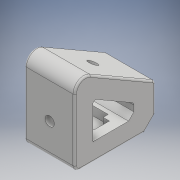
# Autodesk Inventor part: triangle_jig
Saved by Autodesk Inventor 2017 (Build 210142000, 142)
## iProperties
Part Number: triangle_jig
Material: 一般
Document SubType Name: Modeling
Designer: taige
Density: 1 g/cm^3
Appearance: 既定
Author: taige
Autodesk Inventor part; units mm, degrees
ref_plane "YZ Plane" through (0, 0, 0) normal (1, 0, 0) x (0, 1, 0)
ref_plane "XZ Plane" through (0, 0, 0) normal (0, 1, 0) x (-1, 0, 0)
ref_plane "XY Plane" through (0, 0, 0) normal (0, 0, 1) x (1, 0, 0)
sketch "スケッチ1" plane through (0, 0, 0) normal (1, 0, 0) x (0, 1, 0)
  line L0 (-20, 24) -> (63.1384, 24)
  line L1 (63.1384, 24) -> (63.1384, -24)
  line L2 (25, -24) -> (-20, -24)
  line L3 (-20, -24) -> (-20, 24)
  line L4 (-20, 24) -> (63.1384, -24)
  line L5 (-20, -24) -> (25, -24)
  line L6 (25, -24) -> (25, -1.9808)
  line L7 (25, 24) -> (-20, 24)
  line L8 (-20, 24) -> (-20, -24)
  point P0 (0, 0)
  dimension "d6" = 24
  dimension "d7" = 48
  dimension "d96" = 45
  dimension "d98" = 83.1384
  constraints: 18 end point, 4 parallel, 2 horizontal, 2 perpendicular, 2 point on line
  measures "d6" distance from line of point (0, 0) L0
  measures "d7" distance of L2.end L0.start
  measures "d96" distance of L7.end L7.start
  measures "d98" distance of L0.start L0.end
extrude "押し出し1" add sketch "スケッチ1" along normal blind 28 contours L4 L6 L2 L3
sketch "スケッチ2" plane through (28, 0, 0) normal (1, 0, 0) x (0, 0, -1)
  line L0 (-6.6795, -10) -> (14, -10)
  line L1 (14, -10) -> (14, 25.8179)
  line L2 (14, 25.8179) -> (-6.6795, 25.8179)
  line L3 (-6.6795, 25.8179) -> (-6.6795, 13)
  line L4 (-24, -20) -> (24, -20) projected
  line L5 (24, -20) -> (24, 25) projected
  line L6 (-6.6795, -10) -> (14, 25.8179)
  line L7 (14, -10) -> (-6.679, -10)
  line L8 (-6.679, -10) -> (-6.679, 13)
  line L9 (6.5996, 13) -> (14, 13)
  line L10 (14, 13) -> (14, -10)
  point P0 (0, 0)
  point P1 (24, 63.1384)
  dimension "d10" = 20.6795
  dimension "d11" = 35.8179
  dimension "d12" = 10
  dimension "d13" = 10
  dimension "d19" = 20.679
  dimension "d75" = 23
  constraints: 18 end point, 4 parallel, 2 horizontal, 2 perpendicular, 2 point on line
  measures "d10" distance of L2.end L1.end
  measures "d11" distance of L1.end L0.end
  measures "d12" distance between parallel lines of L0 L4
  measures "d13" distance between parallel lines of L5 L1
  measures "d19" distance of L8.end L9.end
  measures "d75" distance between parallel lines of L9 L0
extrude "押し出し2" cut sketch "スケッチ2" against normal blind 40 contours L6 L9 L1 L0
sketch "スケッチ3" plane through (28, -10, 6.6795) normal (0, 1, 0) x (1, 0, 0)
  line L0 (0, 20.6795) -> (0, 0) projected
  line L1 (0, 20.6795) -> (-28, 20.6795) projected
  line L2 (-19.1, 5.5795) -> (-8.9, 5.5795)
  line L3 (-8.9, 5.5795) -> (-8.9, 19.7795)
  line L4 (-8.9, 19.7795) -> (-19.1, 19.7795)
  line L5 (-19.1, 19.7795) -> (-19.1, 5.5795)
  line L6 (-22.6, 8.4295) -> (-5.4, 8.4295)
  line L7 (-5.4, 8.4295) -> (-5.4, 16.9295)
  line L8 (-5.4, 16.9295) -> (-22.6, 16.9295)
  line L9 (-22.6, 16.9295) -> (-22.6, 8.4295)
  point P0 (-28, 6.6795)
  point P1 (-14, 12.6795)
  dimension "d16" = 14
  dimension "d17" = 8
  dimension "d21" = 10.2
  dimension "d22" = 14.2
  dimension "d23" = 7.1
  dimension "d24" = 5.1
  dimension "d25" = 17.2
  dimension "d26" = 8.5
  dimension "d27" = 4.25
  dimension "d28" = 8.6
  constraints: 16 end point, 4 parallel, 2 horizontal, 2 perpendicular
  measures "d16" distance from line of point (-14, 12.679) L0
  measures "d17" distance from line of L1 point (-14, 12.679)
  measures "d21" distance of L4.end L3.end
  measures "d22" distance of L3.end L2.end
  measures "d23" distance from line of point (-14, 12.679) L4
  measures "d24" distance from line of point (-14, 12.679) L5
  measures "d25" distance of L8.end L7.end
  measures "d26" distance of L7.end L6.end
  measures "d27" distance from line of point (-14, 12.679) L8
  measures "d28" distance from line of L9 point (-14, 12.679)
extrude "押し出し3" cut sketch "スケッチ3" against normal blind 5
sketch "スケッチ4" plane through (28, -15, 6.6795) normal (0, 1, 0) x (1, 0, 0)
  line L0 (0, 20.6795) -> (-28, 20.6795) projected
  line L1 (0, 20.6795) -> (0, 0) projected
  circle A0 centre (-14, 12.6795) radius 2.6
  point P0 (-28, 6.6795)
  dimension "d31" = 8
  dimension "d32" = 14
  dimension "d33" = 5.2
  constraints: 1 centre point, 1 coincident
  measures "d31" distance from line of point (-14, 12.679) L0
  measures "d32" distance from line of point (-14, 12.679) L1
  measures "d33" diameter of A0
extrude "押し出し4" cut sketch "スケッチ4" against normal blind 5
fillet "フィレット1" radius 1 4 edges at (8.9, -12.5, -10.25) (8.9, -12.5, -1.75) (19.1, -12.5, -10.25) (19.1, -12.5, -1.75)
sketch "スケッチ8" plane through (28, 25.8179, -14) normal (0, -0.5, -0.866) x (-1, 0, 0)
  line L0 (0, -41.359) -> (28, -41.359) projected
  line L1 (5.4, -35.109) -> (22.6, -35.109)
  line L2 (22.6, -35.109) -> (22.6, -26.609)
  line L3 (22.6, -26.609) -> (5.4, -26.609)
  line L4 (5.4, -26.609) -> (5.4, -35.109)
  line L5 (28, -14.8009) -> (28, -41.359) projected
  line L6 (8.9, -37.959) -> (19.1, -37.959)
  line L7 (19.1, -37.959) -> (19.1, -23.759)
  line L8 (19.1, -23.759) -> (8.9, -23.759)
  line L9 (8.9, -23.759) -> (8.9, -37.959)
  point P0 (28, -29.359)
  point P1 (14, -30.859)
  dimension "d54" = 10.5
  dimension "d55" = 17.2
  dimension "d56" = 8.5
  dimension "d57" = 14
  dimension "d58" = 8.6
  dimension "d59" = 4.25
  dimension "d60" = 10.2
  dimension "d61" = 14.2
  dimension "d62" = 7.1
  dimension "d63" = 5.1
  constraints: 16 end point, 4 parallel, 2 horizontal, 2 perpendicular
  measures "d54" distance from line of point (14, -30.859) L0
  measures "d55" distance of L3.end L2.end
  measures "d56" distance of L2.end L1.end
  measures "d57" distance from line of point (14, -30.859) L5
  measures "d58" distance from line of point (14, -30.859) L2
  measures "d59" distance from line of point (14, -30.859) L3
  measures "d60" distance of L8.end L7.end
  measures "d61" distance of L7.end L6.end
  measures "d62" distance from line of point (14, -30.859) L6
  measures "d63" distance from line of L9 point (14, -30.859)
extrude "押し出し7" cut sketch "スケッチ8" against normal blind 5
sketch "スケッチ9" plane through (28, 28.3179, -9.6699) normal (0, -0.5, -0.866) x (-1, 0, 0)
  line L0 (0, -41.359) -> (28, -41.359) projected
  line L1 (28, -14.8009) -> (28, -41.359) projected
  circle A0 centre (14, -30.859) radius 2.6
  point P0 (28, -29.359)
  point P1 (28, 0)
  dimension "d66" = 10.5
  dimension "d67" = 14
  dimension "d68" = 5.2
  constraints: 1 centre point, 1 coincident
  measures "d66" distance from line of L0 point (14, -30.859)
  measures "d67" distance from line of point (14, -30.859) L1
  measures "d68" diameter of A0
extrude "押し出し8" cut sketch "スケッチ9" against normal blind 5
fillet "フィレット2" radius 1 4 edges at (19.1, -3.3368, 5.7204) (19.1, 4.0244, 1.4704) (8.9, -3.3368, 5.7204) (8.9, 4.0244, 1.4704)
fillet "フィレット4" radius 1.5 1 edges at (14, -10, 6.6795)
sketch "スケッチ10" plane through (0, 13, -14) normal (0, 0, 1) x (1, 0, 0)
  line L0 (0, -23) -> (0, 0) projected
  line L1 (28, -23) -> (0, -23) projected
  line L2 (22.6, -8.25) -> (5.4, -8.25)
  line L3 (5.4, -8.25) -> (5.4, -16.75)
  line L4 (5.4, -16.75) -> (22.6, -16.75)
  line L5 (22.6, -16.75) -> (22.6, -8.25)
  line L6 (19.1, -5.4) -> (8.9, -5.4)
  line L7 (8.9, -5.4) -> (8.9, -19.6)
  line L8 (8.9, -19.6) -> (19.1, -19.6)
  line L9 (19.1, -19.6) -> (19.1, -5.4)
  point P0 (0, -13)
  point P1 (14, -12.5)
  point P2 (0, -22.5)
  dimension "d76" = 14
  dimension "d77" = 10.5
  dimension "d78" = 17.2
  dimension "d79" = 8.5
  dimension "d80" = 8.6
  dimension "d81" = 4.25
  dimension "d82" = 10.2
  dimension "d83" = 14.2
  dimension "d84" = 7.1
  dimension "d85" = 5.1
  constraints: 16 end point, 4 parallel, 2 horizontal, 2 perpendicular
  measures "d76" distance from line of point (14, -12.5) L0
  measures "d77" distance from line of point (14, -12.5) L1
  measures "d78" distance of L4.end L3.end
  measures "d79" distance of L3.end L2.end
  measures "d80" distance from line of point (14, -12.5) L3
  measures "d81" distance from line of point (14, -12.5) L2
  measures "d82" distance of L8.end L7.end
  measures "d83" distance of L7.end L6.end
  measures "d84" distance from line of point (14, -12.5) L6
  measures "d85" distance from line of point (14, -12.5) L7
extrude "押し出し9" cut sketch "スケッチ10" against normal blind 5
sketch "スケッチ11" plane through (0, 13, -19) normal (0, 0, 1) x (1, 0, 0)
  line L0 (28, -23) -> (0, -23) projected
  line L1 (0, -23) -> (0, 0) projected
  circle A0 centre (14, -12.5) radius 2.6
  point P0 (0, -13)
  dimension "d88" = 10.5
  dimension "d89" = 14
  dimension "d90" = 5.2
  constraints: 1 centre point, 1 coincident
  measures "d88" distance from line of point (14, -12.5) L0
  measures "d89" distance from line of point (14, -12.5) L1
  measures "d90" diameter of A0
extrude "押し出し10" cut sketch "スケッチ11" against normal blind 5
fillet "フィレット6" radius 0.5 1 edges at (14, -10, -14)
fillet "フィレット8" radius 2 1 edges at (14, 13, -6.5996)
chamfer "面取り1" distance 6 angle 45 1 edges at (14, 25, -24)
fillet "フィレット9" radius 6 1 edges at (14, -20, 24)
fillet "フィレット10" radius 3 1 edges at (14, -20, -24)
fillet "フィレット11" radius 2 1 edges at (14, 25, -1.9808)
chamfer "面取り3" distance 3 angle 45 1 edges at (14, 13, -14)
fillet "フィレット12" radius 1 7 edges at (0, -17, 18.8038) (0, -20, -3.6962) (0, -19.1213, -23.1213) (0, 1, -24) (0, 24.7321, -2.1355) (0, 25, -10.5677) (0, 6.5, 8.7002)
fillet "フィレット13" radius 1 5 edges at (0.2929, 24.7071, -18.2929) (14.5, 25, -18) (0.2929, 19.2929, -23.7071) (14.5, 19, -24) (0, 22, -21)
fillet "フィレット14" radius 1 10 edges at (28, -17, 18.8038) (28, -20, -3.6962) (28, -19.1213, -23.1213) (28, 0.7929, -24) (28, 18.9685, -23.9239) (28, 22, -21) (28, 24.9239, -17.9685) (28, 25, -10.3606) (28, 24.7321, -2.1355) (28, 6.5, 8.7002)
